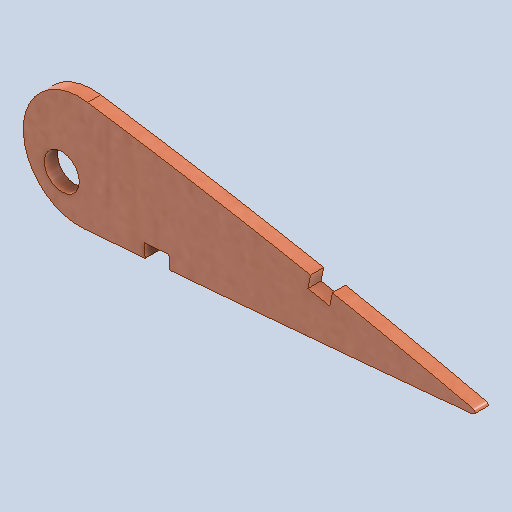
# Autodesk Inventor part: 2P.03.01.09.IM.FlapRibEnd
Saved by Autodesk Inventor 2025.2 (Build 292293000, 293)
## iProperties
Created: 2025-01-05
Part Number: 2P.03.01.09.IM.FlapRibEnd
Material: Wood (Walnut)
Document SubType Name: Modeling
Designer: Imist
Density: 0.55 g/cm^3
Appearance: Walnut - Natural Polished
Author: Imist
Autodesk Inventor part; units mm, degrees
ref_plane "YZ Plane" through (0, 0, 0) normal (1, 0, 0) x (0, 1, 0)
ref_plane "XZ Plane" through (0, 0, 0) normal (0, 1, 0) x (-1, 0, 0)
ref_plane "XY Plane" through (0, 0, 0) normal (0, 0, 1) x (1, 0, 0)
sketch "Sketch1" plane through (0, 0, 0) normal (0, 0, 1) x (1, 0, 0)
  line L0 (18.8258, 8.2146) -> (18.2459, 5.2712)
  line L1 (13.8258, 9.1997) -> (18.8258, 8.2146)
  line L2 (13.2459, 6.2563) -> (13.8258, 9.1997)
  line L3 (18.2459, 5.2712) -> (13.2459, 6.2563)
  spline S0 degree 4 poles (-37.0536, 17.8985) (-31.9132, 17.1283) (-23.3374, 15.8227) (-12.0164, 13.952) (1.6833, 11.5136) (12.6703, 9.4495) (22.4286, 7.5004) (30.8762, 5.7811) (37.8566, 4.2164) (44.6668, 2.844) (48.6838, 1.6374) (51.2021, 1.5715) (51.5064, 0.7295) knots 0 0 0 0 0 0.183688 0.302378 0.416104 0.523956 0.624947 0.717922 0.80148 0.87369 1 1 1 1 1
  spline S1 degree 2 poles (-25.4832, 9.8892) (-25.3745, 9.8731) (-25.2658, 9.857) knots 0 0 0 1 1 1
  line L4 (-25.288, 9.8603) -> (-25.2437, 9.8537) construction
  arc A0 (-25.2481, 9.8544) -> (-25.2836, 9.8596) centre (-40.8454, -94.9669) ccw construction
  line L5 (-24.1701, -3.3757) -> (-23.9226, -6.3655)
  line L6 (-23.9226, -6.3655) -> (-18.2567, -5.8963)
  line L7 (-18.5043, -2.9066) -> (-24.1701, -3.3757)
  line L8 (-38.9493, 5.246) -> (-38.9493, 1.246)
  line L9 (-38.9493, 1.246) -> (-42.9493, 1.246)
  circle A1 centre (-42.9493, 1.246) radius 4
  arc A2 (-37.0536, 17.8985) -> (-37.9116, -7.5055) centre (-38.9493, 5.246) ccw
  line L10 (-18.2567, -5.8963) -> (-18.5043, -2.9066)
  line L11 (-20.2449, -6.0621) -> (-16.2685, -5.7306) construction
  arc A3 (-19.8473, -6.0287) -> (-16.6662, -5.7635) centre (-448.7094, 5192.5355) ccw construction
  spline S2 degree 4 poles (-37.9116, -7.5055) (-32.9709, -7.1034) (-27.9645, -6.6996) (-23.0652, -6.2972) (-18.2567, -5.8963) knots 0 0 0 0 0 1 1 1 1 1
  spline S3 degree 4 poles (9.5327, -3.5271) (11.5362, -3.3527) (15.9784, -2.9631) (22.4725, -2.3822) (30.437, -1.6876) (37.5387, -0.9836) (44.4552, -0.4713) (48.5891, 0.2001) (51.0913, -0.0596) (51.5064, 0.7295) knots 0.442408 0.442408 0.442408 0.442408 0.442408 0.523404 0.624432 0.717481 0.801136 0.873452 1 1 1 1 1
  line L12 (4.8603, -3.9339) -> (14.2051, -3.1204) construction
  arc A4 (5.7946, -3.8508) -> (13.2705, -3.2) centre (-353.3588, 4165.0638) ccw construction
  line L13 (-18.2567, -5.8963) -> (-10.7368, -5.2737) construction
  line L14 (-10.7368, -5.2737) -> (1.5027, -4.2602) construction
  line L15 (1.5027, -4.2602) -> (12.6504, -3.2545) construction
  spline S4 degree 3 poles (-18.2567, -5.8963) (-10.7368, -5.2737) (1.5027, -4.2602) (12.6504, -3.2545) knots 1 1 1 1 2 2 2 2
  point P0 (1.0416, 3.4084)
  point P1 (-2.4286, 1.7343)
  point P2 (-23.0646, 15.7415)
  point P3 (-9.9126, 13.5515)
  point P4 (2.2524, 11.3855)
  point P5 (13.3074, 9.3005)
  point P6 (23.1324, 7.3505)
  point P7 (31.6224, 5.5895)
  point P8 (38.6934, 4.0655)
  point P9 (44.2674, 2.8295)
  point P10 (48.2934, 1.9175)
  point P11 (50.7234, 1.3595)
  point P12 (31.1964, -1.5985)
  point P13 (38.3844, -0.9415)
  point P14 (44.0604, -0.4135)
  point P15 (48.1644, -0.0265)
  point P16 (50.6454, 0.2105)
  point P17 (-51.7356, 5.6816)
  point P18 (51.5064, 1.1705)
  point P19 (-51.7356, 19.9655)
  point P20 (-52.5456, -8.6665)
  point P21 (51.5064, 0.2885)
  point P22 (-37.0536, 5.2315)
  point P23 (-23.0646, 4.7238)
  point P24 (-9.9126, 4.1787)
  point P25 (2.2524, 3.6151)
  point P26 (13.3074, 3.0521)
  point P27 (23.1324, 2.5121)
  point P28 (31.6224, 2.015)
  point P29 (38.6934, 1.5764)
  point P30 (44.2674, 1.2178)
  point P31 (48.2934, 0.9517)
  point P32 (50.7234, 0.7885)
  point P33 (-25.8264, -0.2724)
  point P34 (9.9408, 3.0216)
  point P35 (-19.8876, 9.0264)
  point P36 (-14.6268, 8.1504)
  point P37 (-9.7608, 7.284)
  point P38 (-5.3388, 6.45)
  point P39 (-1.4088, 5.67)
  point P40 (1.9872, 4.9656)
  point P41 (4.8156, 4.356)
  point P42 (7.0452, 3.8616)
  point P43 (8.6556, 3.4968)
  point P44 (9.6276, 3.2736)
  point P45 (-20.2308, 0.1836)
  point P46 (-14.9568, 0.624)
  point P47 (-10.062, 1.0416)
  point P48 (-5.6016, 1.428)
  point P49 (-1.6272, 1.7796)
  point P50 (1.8168, 2.0904)
  point P51 (4.692, 2.3532)
  point P52 (6.9624, 2.5644)
  point P53 (8.604, 2.7192)
  point P54 (9.5964, 2.814)
  point P55 (9.5327, -3.5271)
  dimension "d11" = 3
  dimension "d12" = 5
  dimension "d13" = 52.7751
  dimension "d14" = 3
  dimension "d15" = 5.6658
  dimension "d16" = 4
  dimension "d17" = 4
  dimension "d18" = 8
  constraints: 26 end point, 6 midpoint, 6 point on circle, 5 centre point, 4 parallel, 3 coincident, 3 perpendicular, 1 point on line, 1 tangent, 1 vertical, 39 other
  measures "d11" distance of L0.start L0.end
  measures "d12" horizontal distance of L0.start L1.start
  measures "d13" horizontal distance of L8.start L1.start
  measures "d14" distance of L10.end L10.start
  measures "d15" horizontal distance of L10.end L7.end
  measures "d16" distance of L8.start L8.end
  measures "d17" distance of L8.end L9.end
  measures "d18" diameter of A1
extrude "Extrusion2" add sketch "Sketch1" along normal blind 3 contours S0 S3 S4 L10 L7 L5 S2 A2 L2 L3 L0
body "Solid2"
